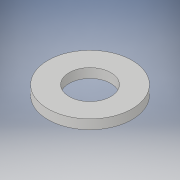
# Autodesk Inventor part: Waher
Saved by Autodesk Inventor 2017.1 (Build 211199000, 199)
## iProperties
Created: 2017-04-20
Part Number: Waher
Material: Generic
Document SubType Name: Modeling
Designer: 196918
Density: 1 g/cm^3
Appearance: Default
Author: 196918
Autodesk Inventor part; units mm, degrees
ref_plane "YZ Plane" through (0, 0, 0) normal (1, 0, 0) x (0, 1, 0)
ref_plane "XZ Plane" through (0, 0, 0) normal (0, 1, 0) x (-1, 0, 0)
ref_plane "XY Plane" through (0, 0, 0) normal (0, 0, 1) x (1, 0, 0)
sketch "Sketch1" plane through (0, 0, 0) normal (0, 1, 0) x (-1, 0, 0)
  circle A0 centre (0, 0) radius 5.6368
  circle A1 centre (0, 0) radius 11.3807
  constraints: 2 centre point, 2 coincident
extrude "Extrusion1" add sketch "Sketch1" along normal blind 2.54
body "Solid1"
